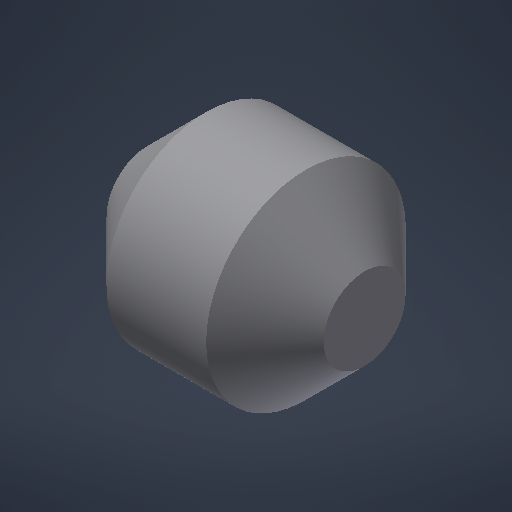
# Autodesk Inventor part: PESAS BAILARINA
Saved by Autodesk Inventor 2026 (Build 300175000, 175)
## iProperties
Created: 2025-03-28
Part Number: PESAS BAILARINA
Material: Generic
Document SubType Name: Modeling
Designer: usuario
Density: 1 g/cm^3
Appearance: Default
Author: usuario
Autodesk Inventor part; units mm, degrees
ref_plane "XZ Plane" through (0, 0, 0) normal (0, 1, 0) x (-1, 0, 0)
ref_plane "XY Plane" through (0, 0, 0) normal (0, 0, 1) x (1, 0, 0)
sketch "Boceto1" plane through (0, 0, 0) normal (1, 0, 0) x (0, 1, 0)
  circle A0 centre (0, 0) radius 7.85
  dimension "d0" = 15.7
  constraints: 1 centre point, 1 coincident
  measures "d0" diameter of A0
ref_plane "Plano de trabajo1" through (11.225, 0, 0) normal (1, 0, 0) x (0, 1, 0)
sketch "Boceto2" plane through (11.225, 0, 0) normal (1, 0, 0) x (0, 1, 0)
  circle A0 centre (0, 0) radius 19.075
  dimension "d2" = 38.15
  constraints: 1 centre point, 1 coincident
  measures "d2" diameter of A0
ref_plane "Plano de trabajo2" through (30.325, 0, 0) normal (1, 0, 0) x (0, 1, 0)
sketch "Boceto3" plane through (30.325, 0, 0) normal (1, 0, 0) x (0, 1, 0)
  point P0 (0, 0)
ref_plane "Plano de trabajo3" through (41.55, 0, 0) normal (1, 0, 0) x (0, 1, 0)
sketch "Boceto4" plane through (41.55, 0, 0) normal (1, 0, 0) x (0, 1, 0)
  circle A0 centre (0, 0) radius 7.85
  dimension "d6" = 15.7
  constraints: 1 centre point, 1 coincident
  measures "d6" diameter of A0
extrude "Extrusión1" add sketch "Boceto2" along normal blind 19.1
extrude "Extrusión2" add sketch "Boceto1" along normal blind 15
extrude "Extrusión3" add sketch "Boceto4" against normal blind 15
loft "Solevación1" add section 1 edges at (41.55, -7.85, 0) section 2 edges at (30.325, -19.075, 0)
loft "Solevación2" add section 1 edges at (0, -7.85, 0) section 2 edges at (11.225, -19.075, 0)
